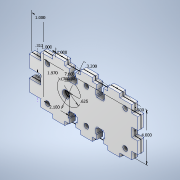
# Autodesk Inventor part: DriveFrame
Saved by Autodesk Inventor 2021 (Build 250183000, 183)
## iProperties
Created: 2021-03-05
Part Number: DriveFrame
Material: Aluminum 6061
Document SubType Name: Modeling
Designer: M3rob
Mass: 704.625 g
Surface Area: 577.588 cm^2
Volume: 260.972 cm^3
Density: 2.7 g/cm^3
Appearance: Aluminum - Flat
Author: M3rob
Autodesk Inventor part; units mm, degrees
ref_plane "YZ Plane" through (0, 0, 0) normal (1, 0, 0) x (0, 1, 0)
ref_plane "XZ Plane" through (0, 0, 0) normal (0, 1, 0) x (-1, 0, 0)
ref_plane "XY Plane" through (0, 0, 0) normal (0, 0, 1) x (1, 0, 0)
sketch "Sketch1" plane through (0, 0, 0) normal (0, 0, 1) x (1, 0, 0)
  line L0 (-96.52, 50.8) -> (-71.12, 50.8)
  line L1 (96.52, 50.8) -> (96.52, 34.925)
  line L2 (96.52, -50.8) -> (71.12, -50.8)
  line L3 (-96.52, -50.8) -> (-96.52, -34.925)
  circle A0 centre (-43.18, 0) radius 40.64 construction
  circle A1 centre (-43.18, 0) radius 7.9375
  circle A2 centre (-43.18, 25.019) radius 2.3813
  circle A3 centre (-43.18, 0) radius 25.019 construction
  circle A4 centre (-60.8711, 17.6911) radius 2.3813
  circle A5 centre (-68.199, 0) radius 2.3813
  circle A6 centre (-60.8711, -17.6911) radius 2.3813
  circle A7 centre (-43.18, -25.019) radius 2.3813
  circle A8 centre (-25.4889, -17.6911) radius 2.3813
  circle A9 centre (-18.161, 0) radius 2.3813
  circle A10 centre (-25.4889, 17.6911) radius 2.3813
  line L4 (-71.12, 50.8) -> (-71.12, 58.7375)
  line L5 (-71.12, 58.7375) -> (-45.72, 58.7375)
  line L6 (-45.72, 58.7375) -> (-45.72, 50.8)
  line L7 (-12.7, 50.8) -> (-12.7, 58.7375)
  line L8 (-12.7, 58.7375) -> (12.7, 58.7375)
  line L9 (12.7, 58.7375) -> (12.7, 50.8)
  line L10 (-45.72, 54.7687) -> (-12.7, 54.7687) construction
  line L11 (45.72, 50.8) -> (45.72, 58.7375)
  line L12 (45.72, 58.7375) -> (71.12, 58.7375)
  line L13 (71.12, 58.7375) -> (71.12, 50.8)
  line L14 (12.7, 54.7687) -> (45.72, 54.7687) construction
  line L15 (71.12, 58.7375) -> (96.52, 50.8) construction
  line L16 (-71.12, 58.7375) -> (-96.52, 50.8) construction
  line L17 (-71.12, -50.8) -> (-71.12, -58.7375)
  line L18 (-71.12, -58.7375) -> (-45.72, -58.7375)
  line L19 (-45.72, -58.7375) -> (-45.72, -50.8)
  line L20 (-12.7, -50.8) -> (-12.7, -58.7375)
  line L21 (-12.7, -58.7375) -> (12.7, -58.7375)
  line L22 (12.7, -58.7375) -> (12.7, -50.8)
  line L23 (45.72, -50.8) -> (45.72, -58.7375)
  line L24 (45.72, -58.7375) -> (71.12, -58.7375)
  line L25 (71.12, -58.7375) -> (71.12, -50.8)
  line L26 (-45.72, 50.8) -> (-12.7, 50.8)
  line L27 (-71.12, 50.8) -> (-45.72, 50.8) construction
  line L28 (-12.7, 50.8) -> (12.7, 50.8) construction
  line L29 (12.7, 50.8) -> (45.72, 50.8)
  line L30 (45.72, 50.8) -> (71.12, 50.8) construction
  line L31 (71.12, 50.8) -> (96.52, 50.8)
  line L32 (71.12, -50.8) -> (45.72, -50.8) construction
  line L33 (45.72, -50.8) -> (12.7, -50.8)
  line L34 (12.7, -50.8) -> (-12.7, -50.8) construction
  line L35 (-12.7, -50.8) -> (-45.72, -50.8)
  line L36 (-45.72, -50.8) -> (-71.12, -50.8) construction
  line L37 (-71.12, -50.8) -> (-96.52, -50.8)
  line L38 (-58.42, 0) -> (58.42, 0) construction
  line L39 (-96.52, 34.925) -> (-121.92, 34.925)
  line L40 (-121.92, 34.925) -> (-121.92, 9.525)
  line L41 (-121.92, 9.525) -> (-96.52, 9.525)
  line L42 (-96.52, -9.525) -> (-121.92, -9.525)
  line L43 (-121.92, -9.525) -> (-121.92, -34.925)
  line L44 (-121.92, -34.925) -> (-96.52, -34.925)
  line L45 (-109.22, 50.8) -> (-109.22, 34.925) construction
  line L46 (-109.22, -34.925) -> (-109.22, -50.8) construction
  line L47 (-96.52, 34.925) -> (-96.52, 50.8)
  line L48 (-96.52, 9.525) -> (-96.52, 34.925) construction
  line L49 (-96.52, -34.925) -> (-96.52, -9.525) construction
  line L50 (-96.52, -9.525) -> (-96.52, 9.525)
  line L51 (96.52, 34.925) -> (109.22, 34.925)
  line L52 (109.22, 34.925) -> (109.22, 9.525)
  line L53 (109.22, 9.525) -> (96.52, 9.525)
  line L54 (96.52, -9.525) -> (109.22, -9.525)
  line L55 (109.22, -9.525) -> (109.22, -34.925)
  line L56 (109.22, -34.925) -> (96.52, -34.925)
  line L57 (96.52, 34.925) -> (96.52, 9.525) construction
  line L58 (96.52, 9.525) -> (96.52, -9.525)
  line L59 (96.52, -9.525) -> (96.52, -34.925) construction
  line L60 (96.52, -34.925) -> (96.52, -50.8)
  point P0 (0, 0)
  point P1 (-96.52, 0)
  point P2 (0, 50.8)
  point P3 (58.42, 58.7375)
  point P4 (-58.42, 58.7375)
  point P5 (0, 0)
  point P6 (-96.52, 0)
  point P7 (96.52, 0)
  dimension "d5" = 50.038
  dimension "d0" = 193.04
  dimension "d1" = 101.6
  dimension "d2" = 81.28
  dimension "d3" = 15.875
  dimension "d4" = 53.34
  dimension "d6" = 4.7625
  dimension "d9" = 360
  dimension "d11" = 25.4
  dimension "d13" = 25.4
  dimension "d14" = 7.9375
  dimension "d15" = 25.4
  dimension "d16" = 12.7
  dimension "d36" = 19.05
  constraints: 122 end point, 119 perpendicular, 76 parallel, 38 point on line, 17 equal length, 11 midpoint, 10 centre point, 10 horizontal, 9 vertical alignment, 8 horizontal alignment, 3 coincident, 3 vertical, 21 other
  measures "d0" distance of L0.start L1.start
  measures "d1" distance of L1.start L2.start
  measures "d2" diameter of A0
  measures "d3" diameter of A1
  measures "d4" distance from line of L3 A0.centre
  measures "d6" diameter of A2
  measures "d11" distance of L4.end L5.end
  measures "d13" distance between parallel lines of L3 L4
  measures "d14" distance between parallel lines of L0 L5
  measures "d15" distance between parallel lines of L3 L40
  measures "d16" distance of L1.end L51.end
  measures "d36" distance between parallel lines of L42 L41
extrude "Extrusion1" add sketch "Sketch1" along normal mid plane 12.7 contours L0 L4 L5 L6 L26 L7 L8 L9 L29 L11 L12 L13 L31 L1 L51 L52 L53 L58 L54 L55 L56 L60 L2 L25 L24 L23 L33 L22 L21 L20 L35 L19 L18 L17 L37 L3 L44 L43 L42 L50 L41 L40 L39 L47 | A2 | A4 | A5 | A6 | A7 | A8 | A9 | A10
sketch "Sketch2" plane through (0, 0, 6.35) normal (0, 0, 1) x (1, 0, 0)
  line L0 (-45.72, 50.8) -> (-12.7, 50.8) construction
  line L1 (-35.9537, 50.8) -> (-35.9537, 41.275)
  line L2 (-35.9537, 41.275) -> (-38.735, 41.275)
  line L3 (-38.735, 41.275) -> (-38.735, 30.1625)
  line L4 (-38.735, 30.1625) -> (-35.9537, 30.1625)
  line L5 (-35.9537, 30.1625) -> (-35.9537, 26.9875)
  line L6 (-35.9537, 26.9875) -> (-22.4663, 26.9875)
  line L7 (-22.4663, 26.9875) -> (-22.4663, 30.1625)
  line L8 (-22.4663, 30.1625) -> (-19.685, 30.1625)
  line L9 (-19.685, 30.1625) -> (-19.685, 41.275)
  line L10 (-19.685, 41.275) -> (-22.4663, 41.275)
  line L11 (-22.4663, 50.8) -> (-22.4663, 41.275)
  line L12 (-35.9537, 50.8) -> (-35.9537, 50.8)
  line L13 (-35.9537, 50.8) -> (-22.4663, 50.8)
  line L14 (-22.4663, 50.8) -> (-22.4663, 50.8)
  line L15 (-29.21, 50.8) -> (-29.21, 26.9875) construction
  line L16 (45.72, 50.8) -> (12.7, 50.8) construction
  line L17 (22.4663, 50.8) -> (22.4663, 41.275)
  line L18 (22.4663, 41.275) -> (19.685, 41.275)
  line L19 (19.685, 41.275) -> (19.685, 30.1625)
  line L20 (19.685, 30.1625) -> (22.4663, 30.1625)
  line L21 (22.4663, 30.1625) -> (22.4663, 26.9875)
  line L22 (22.4663, 26.9875) -> (35.9537, 26.9875)
  line L23 (35.9537, 26.9875) -> (35.9537, 30.1625)
  line L24 (35.9537, 30.1625) -> (38.735, 30.1625)
  line L25 (38.735, 30.1625) -> (38.735, 41.275)
  line L26 (38.735, 41.275) -> (35.9537, 41.275)
  line L27 (35.9537, 50.8) -> (22.4663, 50.8)
  line L28 (35.9537, 50.8) -> (35.9537, 41.275)
  line L29 (29.21, 50.8) -> (29.21, 26.9875) construction
  line L30 (-96.52, 9.525) -> (-96.52, -9.525) construction
  line L31 (-96.52, 0) -> (96.52, 0) construction
  line L32 (96.52, -9.525) -> (96.52, 9.525) construction
  line L33 (-35.9537, -50.8) -> (-35.9537, -41.275)
  line L34 (-35.9537, -41.275) -> (-38.735, -41.275)
  line L35 (-38.735, -41.275) -> (-38.735, -30.1625)
  line L36 (-38.735, -30.1625) -> (-35.9537, -30.1625)
  line L37 (-35.9537, -30.1625) -> (-35.9537, -26.9875)
  line L38 (-35.9537, -26.9875) -> (-22.4663, -26.9875)
  line L39 (-22.4663, -26.9875) -> (-22.4663, -30.1625)
  line L40 (-22.4663, -30.1625) -> (-19.685, -30.1625)
  line L41 (-19.685, -30.1625) -> (-19.685, -41.275)
  line L42 (-19.685, -41.275) -> (-22.4663, -41.275)
  line L43 (-22.4663, -50.8) -> (-22.4663, -41.275)
  line L44 (-35.9537, -50.8) -> (-22.4663, -50.8)
  line L45 (-29.21, -50.8) -> (-29.21, -26.9875) construction
  line L46 (22.4663, -50.8) -> (22.4663, -41.275)
  line L47 (22.4663, -41.275) -> (19.685, -41.275)
  line L48 (19.685, -41.275) -> (19.685, -30.1625)
  line L49 (19.685, -30.1625) -> (22.4663, -30.1625)
  line L50 (22.4663, -30.1625) -> (22.4663, -26.9875)
  line L51 (22.4663, -26.9875) -> (35.9537, -26.9875)
  line L52 (35.9537, -26.9875) -> (35.9537, -30.1625)
  line L53 (35.9537, -30.1625) -> (38.735, -30.1625)
  line L54 (38.735, -30.1625) -> (38.735, -41.275)
  line L55 (38.735, -41.275) -> (35.9537, -41.275)
  line L56 (35.9537, -50.8) -> (22.4663, -50.8)
  line L57 (35.9537, -50.8) -> (35.9537, -41.275)
  line L58 (29.21, -50.8) -> (29.21, -26.9875) construction
  point P0 (0, 0)
  dimension "d19" = 13.4874
  dimension "d20" = 9.525
  dimension "d21" = 3.175
  dimension "d22" = 11.1125
  dimension "d23" = 19.05
  constraints: 110 end point, 37 point on line, 31 symmetric about line, 14 perpendicular, 8 midpoint, 5 equal length, 3 vertical, 2 collinear, 1 coincident, 1 parallel, 2 other
  measures "d19" distance between parallel lines of L12 L14
  measures "d20" distance between parallel lines of L0 L2
  measures "d21" distance between parallel lines of L4 L6
  measures "d22" distance of L2.end L3.end
  measures "d23" distance between parallel lines of L9 L3
extrude "Extrusion2" cut sketch "Sketch2" against normal through all
sketch "Sketch3" plane through (0, 0, 6.35) normal (0, 0, 1) x (1, 0, 0)
  circle A0 centre (-82.4376, 36.7176) radius 14.0824 construction
  circle A1 centre (82.4376, 36.7176) radius 14.0824 construction
  circle A2 centre (82.4376, -36.7176) radius 14.0824 construction
  circle A3 centre (-82.4376, -36.7176) radius 14.0824 construction
  line L0 (-71.12, 50.8) -> (-96.52, 50.8) construction
  line L1 (-96.52, 50.8) -> (-96.52, 34.925) construction
  line L2 (-96.52, -50.8) -> (-71.12, -50.8) construction
  line L3 (-96.52, -34.925) -> (-96.52, -50.8) construction
  line L4 (96.52, 34.925) -> (96.52, 50.8) construction
  line L5 (96.52, 50.8) -> (71.12, 50.8) construction
  line L6 (96.52, -50.8) -> (96.52, -34.925) construction
  line L7 (71.12, -50.8) -> (96.52, -50.8) construction
  circle A4 centre (-82.4376, 36.7176) radius 4.7625 construction
  line L8 (-83.82, 50.8) -> (-83.82, 41.275) construction
  circle A5 centre (0, 36.7176) radius 14.0824 construction
  circle A6 centre (0, -36.7176) radius 14.0824 construction
  point P0 (0, 0)
  dimension "d34" = 9.525
  dimension "d35" = 9.525
  constraints: 8 tangent, 6 centre point, 5 equal radius, 2 end point, 2 horizontal alignment, 2 vertical alignment, 1 coincident, 1 midpoint, 1 perpendicular, 3 other
  measures "d35" distance of L8.start L8.end
hole "Hole1" at (-82.4376, 36.7176, 6.35) at (82.4376, 36.7176, 6.35) at (82.4376, -36.7176, 6.35) at (-82.4376, -36.7176, 6.35) at (0, 36.7176, 6.35) at (0, -36.7176, 6.35) direction (0, 0, -1) diameter 10.0838 depth 35.179 tip angle 118 clearance for "Hex Head Bolt" size "3/8" standard "Ansi Unified Screw Threads"
body "Solid1"
